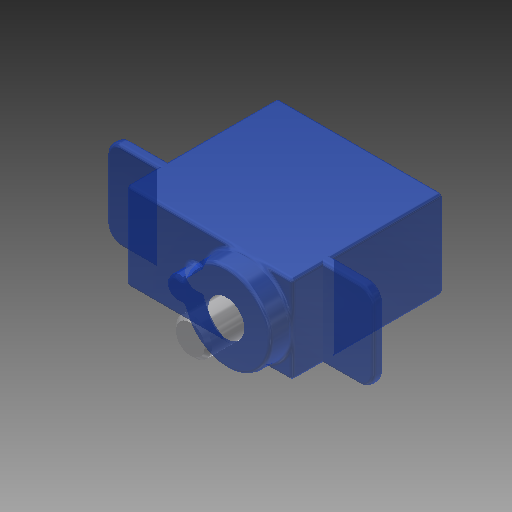
# Autodesk Inventor part: towerpro sg90
Saved by Autodesk Inventor 2018 (Build 220112000, 112)
## iProperties
Created: 2012-04-10
Part Number: towerpro sg90
Document SubType Name: Modeling
Designer: Darcy
Density: 1 g/cm^3
Material: Generic
Appearance: Clear - Blue
Author: Darcy
Autodesk Inventor part; units mm, degrees
ref_plane "YZ Plane" through (0, 0, 0) normal (1, 0, 0) x (0, 1, 0)
ref_plane "XZ Plane" through (0, 0, 0) normal (0, 1, 0) x (-1, 0, 0)
sketch "Sketch1" plane through (0, 0, 0) normal (0, 0, 1) x (1, 0, 0)
  line L0 (0, 0) -> (23, 0)
  line L1 (23, 0) -> (23, -12.2)
  line L2 (23, -12.2) -> (0, -12.2)
  line L3 (0, -12.2) -> (0, 0)
  dimension "d0" = 23
  dimension "d1" = 12.2
  constraints: 8 end point, 2 parallel, 1 horizontal, 1 perpendicular
  measures "d0" distance of L1.end L2.end
  measures "d1" distance of L2.end L0.start
extrude "Extrusion1" add sketch "Sketch1" along normal blind 29
sketch "Sketch2" plane through (0, 0, 29) normal (0, 0, 1) x (1, 0, 0)
  line L0 (23, 0) -> (23, -12.2) projected
  line L1 (0, 0) -> (23, 0) projected
  line L2 (0, -12.2) -> (0, 0) projected
  line L3 (23, -12.2) -> (0, -12.2) projected
  circle A0 centre (16.9, -6.1) radius 6.1
  circle A1 centre (10, -6.1) radius 1.5
  dimension "d4" = 6.9
  dimension "d5" = 3
  dimension "d6" = 6.1
  constraints: 3 tangent, 2 centre point
  measures "d4" distance of A0.centre A1.centre
  measures "d5" diameter of A1
  measures "d6" distance from line of L1 A1.centre
extrude "Extrusion2" cut sketch "Sketch2" against normal blind 8 contours L0 A0 L1 | L0 L3 A0 | A0 A1 L3 L2 L1
sketch "Sketch3" plane through (0, 0, 29) normal (0, 0, 1) x (1, 0, 0)
  arc A0 (10.916667, -7.287317) -> (10.916667, -4.912683) centre (16.9, -6.1) ccw
  arc A1 (10.916667, -4.912683) -> (10.916667, -7.287317) centre (10, -6.1) ccw
  circle A2 centre (16.9, -6.1) radius 2.5
  point P0 (0, 0)
  dimension "d9" = 5
  constraints: 1 centre point, 1 coincident
  measures "d9" diameter of A2
extrude "Extrusion3" cut sketch "Sketch3" against normal blind 5
ref_plane "Work Plane1" through (0, 0, 16) normal (0, 0, 1) x (1, 0, 0)
sketch "Sketch4" plane through (0, 0, 16) normal (0, 0, 1) x (1, 0, 0)
  line L0 (0, 0) -> (23, 0) projected
  line L1 (23, 0) -> (23, -12.2) projected
  line L2 (23, -12.2) -> (0, -12.2) projected
  line L3 (0, -12.2) -> (0, 0) projected
  line L4 (30, -12.2) -> (-7, -12.2)
  line L5 (-7, -12.2) -> (-7, 0)
  line L6 (-7, 0) -> (30, 0)
  line L7 (30, 0) -> (30, -12.2)
  dimension "d13" = 12.2
  dimension "d14" = 7
  dimension "d15" = 7
  constraints: 8 end point, 2 parallel, 1 horizontal, 1 perpendicular, 1 point on line
  measures "d13" distance of L6.end L4.start
  measures "d14" distance between parallel lines of L1 L7
  measures "d15" distance between parallel lines of L3 L5
extrude "Extrusion4" add sketch "Sketch4" along normal mid plane 1.5 contours L3 L4 L5 L6 | L6 L7 L4 L1
fillet "Fillet1" radius 0.5 16 edges at (8.5, -6.1, 24) (10.9167, -4.9127, 22.5) (8.5, -6.1, 21) (10.9167, -7.2873, 22.5) (23, -6.1, 24) (13.0291, -10.8145, 21) (21.2134, -10.4134, 21) (21.2134, -1.7866, 21) (13.0291, -1.3855, 21) (19.95, -12.2, 21) (23, -9.15, 21) (23, -3.05, 21) (19.95, 0, 21) (8.45, 0, 21) (0, -6.1, 21) (8.45, -12.2, 21)
fillet "Fillet2" radius 2 4 edges at (-7, -12.2, 16) (-7, 0, 16) (30, -12.2, 16) (30, 0, 16)
fillet "Fillet3" radius 0.5 44 edges at (23, -12.2, 18.625) (0, -12.2, 18.625) (0, -12.2, 7.625) (11.5, -12.2, 0) (23, -12.2, 6.2531) (23, -12.2, 13.2242) (23, -12.2, 14.5961) (23, 0, 18.625) (23, -6.1, 0) (23, 0, 6.2531) (23, 0, 13.2242) (23, 0, 14.5961) (0, 0, 7.625) (0, -6.1, 0) (0, 0, 18.625) (11.5, 0, 0) (22.8536, -12.0536, 20.8536) (0.1464, -12.0536, 20.8536) (22.8536, -0.1464, 20.8536) (0.1464, -0.1464, 20.8536) (30, -6.1, 16.75) (30, -6.1, 15.25) (23.4789, 0, 16.75) (25.9789, 0, 16.75) (25.9789, -12.2, 16.75) (23.4789, -12.2, 16.75) (25.9789, -12.2, 15.25) (23.4789, -12.2, 15.25) (23.4789, 0, 15.25) (25.9789, 0, 15.25) (-2.5, -12.2, 16.75) (-2.5, -12.2, 15.25) (-7, -6.1, 15.25) (-7, -6.1, 16.75) (-2.5, 0, 15.25) (-2.5, 0, 16.75) (29.4142, -11.6142, 16.75) (29.4142, -0.5858, 16.75) (29.4142, -0.5858, 15.25) (29.4142, -11.6142, 15.25) (-6.4142, -11.6142, 16.75) (-6.4142, -0.5858, 16.75) (-6.4142, -11.6142, 15.25) (-6.4142, -0.5858, 15.25)
chamfer "Chamfer1" distance 0.5 angle 45 1 edges at (14.4, -6.1, 29)
body "Solid1"
